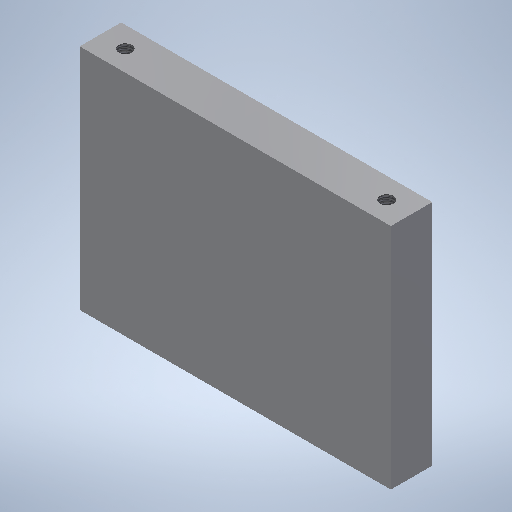
# Autodesk Inventor part: Sides
Saved by Autodesk Inventor 2025 (Build 290162000, 162)
## iProperties
Created: 2010-12-14
Part Number: Sides
Document SubType Name: Modeling
Designer: berny
Density: 2.7 g/cm^3
Material: Aluminum-6061
Mass: 209.739 g
Surface Area: 207.587 cm^2
Volume: 77.6811 cm^3
Appearance: Aluminum - Flat
Author: berny
Autodesk Inventor part; units mm, degrees
ref_plane "YZ Plane" through (0, 0, 0) normal (1, 0, 0) x (0, 1, 0)
ref_plane "XZ Plane" through (0, 0, 0) normal (0, 1, 0) x (-1, 0, 0)
ref_plane "XY Plane" through (0, 0, 0) normal (0, 0, 1) x (1, 0, 0)
sketch "Sketch1" plane through (0, 0, 0) normal (0, 0, 1) x (1, 0, 0)
  line L0 (0, 0) -> (75, 0)
  line L1 (75, 0) -> (75, 55)
  line L2 (75, 55) -> (0, 55)
  line L3 (0, 55) -> (0, 0)
  dimension "d0" = 55
  dimension "d1" = 75
  constraints: 8 end point, 2 parallel, 1 horizontal, 1 perpendicular
  measures "d0" distance of L2.end L0.start
  measures "d1" distance of L0.start L0.end
extrude "Extrusion1" add sketch "Sketch1" along normal blind 10
sketch "Sketch3" plane through (0, 0, 0) normal (0, -1, 0) x (1, 0, 0)
  line L0 (0, 0) -> (0, 10) projected
  line L1 (0, 0) -> (75, 0) projected
  line L2 (75, 0) -> (75, 10) projected
  point P0 (6, 5)
  point P1 (69, 5)
  dimension "d14" = 6
  dimension "d15" = 6
  dimension "d16" = 5
  constraints: 1 horizontal alignment
  measures "d14" distance from line of L2 point (69, 5)
  measures "d15" distance from line of L0 point (6, 5)
  measures "d16" distance from line of L1 point (6, 5)
hole "Hole2" at (6, 0, 5) at (69, 0, 5) direction (0, 1, 0) diameter 3.242 depth 11.8 tip angle 118 thread size "M4x0.7" class "6H" standard "ANSI Metric M Profile"
sketch "Sketch4" plane through (0, 55, 0) normal (0, 1, 0) x (1, 0, 0)
  line L0 (75, 0) -> (75, -10) projected
  line L1 (75, 0) -> (0, 0) projected
  line L2 (0, 0) -> (0, -10) projected
  point P0 (6, -5)
  point P1 (69, -5)
  dimension "d24" = 5
  dimension "d25" = 6
  dimension "d26" = 6
  constraints: 1 horizontal alignment
  measures "d24" distance from line of L1 point (6, -5)
  measures "d25" distance from line of point (6, -5) L2
  measures "d26" distance from line of L0 point (69, -5)
hole "Hole3" at (6, 55, 5) at (69, 55, 5) direction (0, -1, 0) diameter 3.242 depth 11.8 tip angle 118 thread size "M4x0.7" class "6H" standard "ANSI Metric M Profile"
equation "\"d26\" = d25"
body "Solid1"
